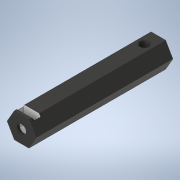
# Autodesk Inventor part: SupportSecondToCoverNew
Saved by Autodesk Inventor 2020 (Build 240168000, 168)
## iProperties
Created: 2018-12-30
Part Number: SupportSecondToCoverNew
Material: ABS Plastic
Document SubType Name: Modeling
Designer: Victor Sabino
Density: 1.06 g/cm^3
Appearance: Smooth - White
Mass: 5.01621 g
Surface Area: 28.6628 cm^2
Volume: 4.73227 cm^3
Author: Victor Sabino
Autodesk Inventor part; units mm, degrees
ref_plane "YZ Plane" through (0, 0, 0) normal (1, 0, 0) x (0, 1, 0)
ref_plane "XZ Plane" through (0, 0, 0) normal (0, 1, 0) x (-1, 0, 0)
ref_plane "XY Plane" through (0, 0, 0) normal (0, 0, 1) x (1, 0, 0)
sketch "Sketch1" plane through (0, 0, 0) normal (0, 0, 1) x (1, 0, 0)
  line L0 (-2.3383, -4.05) -> (-4.6765, 0)
  line L1 (-4.6765, 0) -> (-2.3383, 4.05)
  line L2 (-2.3383, 4.05) -> (2.3383, 4.05)
  line L3 (2.3383, 4.05) -> (4.6765, 0)
  line L4 (4.6765, 0) -> (2.3383, -4.05)
  line L5 (2.3383, -4.05) -> (-2.3383, -4.05)
  point P0 (0, 0)
  point P1 (0, 0)
  dimension "d0" = 4.05
  constraints: 12 end point, 1 coincident, 13 other
  measures "d0" distance from line of L5 point (0, 0)
extrude "Extrusion1" add sketch "Sketch1" against normal blind 44
sketch "Sketch2" plane through (4.6765, 0, 0) normal (0.8660254, 0.5, 0) x (0, 0, -1)
  line L0 (0, 4.6765) -> (0, 0) projected
  line L1 (4.75, 5.1383) -> (7.25, 5.1383)
  line L2 (7.25, 5.1383) -> (7.25, -0.4617)
  line L3 (7.25, -0.4617) -> (4.75, -0.4617)
  line L4 (4.75, -0.4617) -> (4.75, 5.1383)
  line L5 (4.75, 5.1383) -> (7.25, -0.4617) construction
  line L6 (7.25, 5.1383) -> (4.75, -0.4617) construction
  point P0 (0, 2.3383)
  point P1 (6, 2.3383)
  dimension "d3" = 2.5
  dimension "d4" = 5.6
  dimension "d10" = 0
  dimension "d11" = 6
  constraints: 12 end point, 2 midpoint, 2 parallel, 1 horizontal, 1 perpendicular
  measures "d3" distance of L2.end L3.end
  measures "d4" distance of L1.end L2.end
  measures "d10" vertical distance of point (0, 2.338) point (6, 2.338)
  measures "d11" horizontal distance of L0.end point (6, 2.338)
extrude "Extrusion2" [suppressed]
sketch "Sketch3" plane through (0, 0, 0) normal (0, 0, 1) x (1, 0, 0)
  circle A0 centre (0, 0) radius 1.5
  dimension "d7" = 3
  constraints: 1 centre point, 1 coincident
  measures "d7" diameter of A0
extrude "Extrusion3" cut sketch "Sketch3" against normal blind 8
ref_plane "Work Plane1" through (0, 0, -22) normal (0, 0, -1) x (-1, 0, 0)
mirror "Mirror1" [suppressed]
sketch "Sketch4" plane through (1.5014, 4.1, -7.25) normal (0, 0, 1) x (1, 0, 0)
  line L0 (0, 0) -> (-4.5469, -2.6251) projected
  line L1 (-1.7469, -7.4749) -> (-4.5469, -2.6251) projected
  line L2 (2.8, -4.8497) -> (-1.7469, -7.4749) projected
  line L3 (-4.5469, -2.6251) -> (-4.5469, -5.8583)
  line L4 (-1.7469, -7.4749) -> (-4.5469, -5.8583)
  line L5 (-1.7469, -7.4749) -> (-4.5469, -2.6251)
  point P0 (-1.5014, -4.1)
  dimension "d12" = 120
  dimension "d13" = 120
  constraints: 6 end point, 1 collinear
  measures "d12" angle of L3 L0
  measures "d13" angle of L2 L4
extrude "Extrusion4" [suppressed]
sketch "Sketch5" plane through (-4.6765, 0, -44) normal (-0.8660254, -0.5, 0) x (0, 0, 1)
  line L0 (0, -4.6765) -> (0, 0) projected
  line L1 (4.75, 0.5197) -> (7.25, 0.5197)
  line L2 (7.25, 0.5197) -> (7.25, -5.0803)
  line L3 (7.25, -5.0803) -> (4.75, -5.0803)
  line L4 (4.75, -5.0803) -> (4.75, 0.5197)
  line L5 (4.75, 0.5197) -> (7.25, -5.0803) construction
  line L6 (7.25, 0.5197) -> (4.75, -5.0803) construction
  line L7 (0, -3.8671) -> (0, -0.8671) projected
  line L8 (0, -4.6765) -> (0, 0) projected
  line L9 (0, 0) -> (0, 2.3383) projected
  line L10 (0, 2.3383) -> (0, 0) projected
  line L11 (0, 0) -> (0, -4.6765) projected
  line L12 (0, -4.6765) -> (0, -7.0148) projected
  line L13 (0, -7.0148) -> (0, -4.6765) projected
  line L14 (9.5, -0.8671) -> (9.5, -3.8671) projected
  line L15 (0, -3.8671) -> (0, -0.8671) projected
  line L16 (44, -7.0148) -> (0, -7.0148) projected
  line L17 (44, 2.3383) -> (0, 2.3383) projected
  point P0 (44, -2.3383)
  point P1 (6, -2.2803)
  dimension "d16" = 2.5
  dimension "d17" = 5.6
  dimension "d18" = 6
  dimension "d25" = 1.9345
  constraints: 12 end point, 2 midpoint, 2 parallel, 1 horizontal, 1 perpendicular
  measures "d16" distance of L2.end L3.end
  measures "d17" distance of L1.end L2.end
  measures "d18" distance from line of L0 point (6, -2.28)
  measures "d25" distance between parallel lines of L16 L3
extrude "Extrusion5" [suppressed]
sketch "Sketch6" plane through (-1.5019, -4.1, -42.75) normal (0, 0, -1) x (-1, 0, 0)
  line L0 (-1.7472, 7.4751) -> (-4.5472, 2.6253) projected
  line L1 (-4.5472, 2.6253) -> (-4.5472, 5.8585)
  line L2 (-1.7472, 7.4751) -> (-4.5472, 5.8585)
  line L3 (2.7993, 4.8501) -> (-1.7472, 7.4751) projected
  line L4 (0, 0) -> (-4.5472, 2.6253) projected
  line L5 (-1.7472, 7.4751) -> (-4.5472, 2.6253)
  point P0 (-1.5019, 4.1)
  dimension "d21" = 120
  dimension "d22" = 120
  constraints: 6 end point, 1 perpendicular
  measures "d21" angle of L3 L2
  measures "d22" angle of L4 L1
extrude "Extrusion6" [suppressed]
sketch "Sketch8" plane through (0, 0, -44) normal (0, 0, -1) x (-1, 0, 0)
  line L0 (-2.8, 1.25) -> (2.8, 1.25)
  line L1 (2.8, 1.25) -> (2.8, -1.25)
  line L2 (2.8, -1.25) -> (-2.8, -1.25)
  line L3 (-2.8, -1.25) -> (-2.8, 1.25)
  circle A0 centre (0, 0) radius 1.5 projected
  line L4 (-2.8, 1.25) -> (2.8, -1.25) construction
  line L5 (2.8, 1.25) -> (-2.8, -1.25) construction
  dimension "d32" = 5.6
  dimension "d33" = 2.5
  constraints: 12 end point, 2 midpoint, 2 parallel, 1 horizontal, 1 perpendicular
  measures "d32" distance of L1.end L2.end
  measures "d33" distance of L0.end L1.end
extrude "Extrusion8" cut sketch "Sketch8" against normal blind 6.5 contours L0 A0 L2 L3 | L0 A0 L2 | L0 L1 L2 A0
sketch "Sketch9" plane through (-2.3383, 4.05, 0) normal (0, 1, 0) x (1, 0, 0)
  line L0 (4.6765, 0) -> (4.6765, 44) projected
  line L1 (0, 44) -> (4.6765, 44) projected
  line L2 (0, 0) -> (0, 44) projected
  line L3 (0, 0) -> (4.6765, 0) projected
  line L4 (5.1383, 44) -> (-0.4617, 44) projected
  line L5 (2.3383, 44) -> (2.3383, 0) construction
  line L6 (2.3383, 44) -> (46.3383, 44) construction
  circle A0 centre (2.3383, 39.5) radius 1.5
  dimension "d36" = 90
  dimension "d37" = 3
  dimension "d38" = 0
  dimension "d39" = 4.5
  constraints: 4 end point, 1 centre point, 1 horizontal, 1 midpoint, 1 perpendicular, 1 vertical
  measures "d36" angle of L5 L6
  measures "d37" diameter of A0
  measures "d38" distance from line of L5 A0.centre
  measures "d39" distance of L5.start A0.centre
extrude "Extrusion9" cut sketch "Sketch9" against normal up to surface (8.1 mm away) contours A0
sketch "Sketch10" plane through (-2.8, 1.25, -44) normal (0, -1, 0) x (1, 0, 0)
  circle A0 centre (2.8, 4.5) radius 1.5 projected
  line L0 (5.6, 0) -> (0, 0) projected
  line L1 (5.6, 0) -> (5.6, 6.5) projected
  line L2 (5.6, 6.5) -> (0, 6.5) projected
  line L3 (0, 0) -> (0, 6.5) projected
  line L4 (0, 6.5) -> (2.8, 8.1166)
  line L5 (0, 6.5) -> (3.9156, 6.5) construction
  line L6 (5.6, 6.5) -> (2.8, 8.1166)
  line L7 (5.6, 6.5) -> (8.8332, 6.5) construction
  line L8 (5.6, 6.5) -> (0, 6.5)
  point P0 (2.8, 44)
  dimension "d42" = 30
  dimension "d43" = 150
  constraints: 10 end point, 2 horizontal, 1 collinear, 1 equal length
  measures "d42" angle of L5 L4
  measures "d43" angle of L7 L6
extrude "Extrusion10" cut sketch "Sketch10" along normal blind 2.5 contours L2 L4 L6
sketch "Sketch11" plane through (-2.3383, 4.05, 0) normal (0, 1, 0) x (1, 0, 0)
  circle A0 centre (2.3383, 39.5) radius 1.5 projected
  line L0 (0, 0) -> (4.6765, 0) projected
  line L1 (4.6765, 0) -> (4.6765, 44) projected
  line L2 (0, 44) -> (4.6765, 44) projected
  line L3 (0, 0) -> (0, 44) projected
  line L4 (-0.4617, 0.8) -> (5.1383, 0.8)
  line L5 (5.1383, 0.8) -> (5.1383, 3.3)
  line L6 (5.1383, 3.3) -> (-0.4617, 3.3)
  line L7 (-0.4617, 3.3) -> (-0.4617, 0.8)
  line L8 (-0.4617, 0.8) -> (5.1383, 3.3) construction
  line L9 (5.1383, 0.8) -> (-0.4617, 3.3) construction
  point P0 (2.3383, 0)
  point P1 (2.3383, 2.05)
  dimension "d46" = 5.6
  dimension "d47" = 2.5
  dimension "d48" = 2.05
  constraints: 12 end point, 2 midpoint, 2 parallel, 1 horizontal, 1 perpendicular
  measures "d46" distance of L6.end L5.end
  measures "d47" distance of L5.end L4.end
  measures "d48" distance of point (2.338, 0) point (2.338, 2.05)
extrude "Extrusion11" cut sketch "Sketch11" against normal blind 5.85 contours L4 L7 L6 L3 | L3 L6 L1 L4 | L1 L6 L5 L4
sketch "Sketch12" plane through (2.3383, 4.05, -0.8) normal (0, 0, -1) x (-1, 0, 0)
  line L0 (5.1383, -0.7997) -> (4.6765, 0) projected
  line L1 (5.1383, -0.7997) -> (5.1383, -5.85) projected
  line L2 (5.1383, -5.85) -> (-0.4617, -5.85) projected
  line L3 (-0.4617, -0.7997) -> (-0.4617, -5.85) projected
  line L4 (0, 0) -> (-0.4617, -0.7997) projected
  line L5 (4.6765, 0) -> (0, 0) projected
  circle A0 centre (2.3383, -4.05) radius 1.5 projected
  line L6 (5.1383, -5.85) -> (2.3383, -7.4666)
  line L7 (5.1383, -5.85) -> (8.4476, -5.85) construction
  line L8 (-0.4617, -5.85) -> (2.3383, -7.4666)
  line L9 (-0.4617, -5.85) -> (2.7714, -5.85) construction
  dimension "d52" = 150
  dimension "d53" = 30
  constraints: 8 end point, 2 horizontal, 1 equal length
  measures "d52" angle of L6 L7
  measures "d53" angle of L8 L9
extrude "Extrusion12" cut sketch "Sketch12" along normal up to surface (2.5 mm away) contours L6 L8 L2
body "Solid1"
